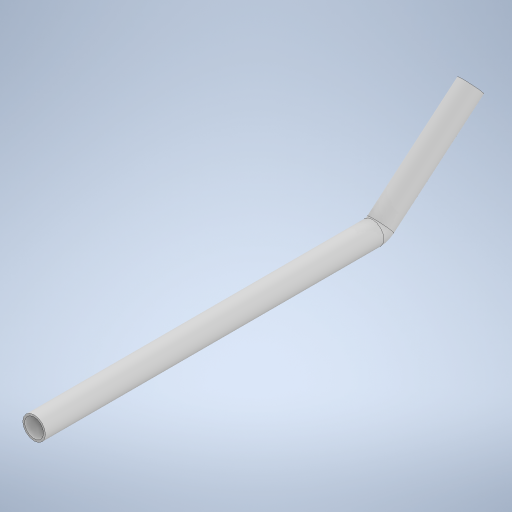
# Autodesk Inventor part: Sit Link 2
Saved by Autodesk Inventor 2024 (Build 280153000, 153)
## iProperties
Created: 2023-10-23
Part Number: Sit Link 2
Material: Generic
Document SubType Name: Modeling
Designer: tinas
Density: 1 g/cm^3
Appearance: Default
Author: tinas
Autodesk Inventor part; units mm, degrees
ref_plane "YZ Plane" through (0, 0, 0) normal (1, 0, 0) x (0, 1, 0)
ref_plane "XY Plane" through (0, 0, 0) normal (0, 0, 1) x (1, 0, 0)
sketch "Sketch1" plane through (0, 0, 0) normal (0, 0, 1) x (1, 0, 0)
  circle A0 centre (0, 0) radius 12
  circle A1 centre (0, 0) radius 10
  dimension "d0" = 24
  dimension "d1" = 20
  constraints: 2 centre point, 2 coincident
  measures "d0" diameter of A0
  measures "d1" diameter of A1
extrude "Extrusion1" add sketch "Sketch1" along normal blind 500
ref_plane "Work Plane1" through (0, -12, 0) normal (0, 1, 0) x (-1, 0, 0)
sketch "Sketch2" plane through (0, -12, 0) normal (0, 1, 0) x (-1, 0, 0)
  line L0 (-136.7178, 142) -> (138.1684, 142)
  line L1 (12, 0) -> (-12, 0) projected
  point P0 (0, 0)
  dimension "d4" = 142
  constraints: 2 end point, 1 horizontal
  measures "d4" distance between parallel lines of L1 L0
bend part "Bend Part1" radius 25.4 angle 40 line through (136.7178, -12, 142) along (-1, 0, 0) centre toward (0, 1, 0) moving side (0, 0, -1) both sides no
body "Solid1"
